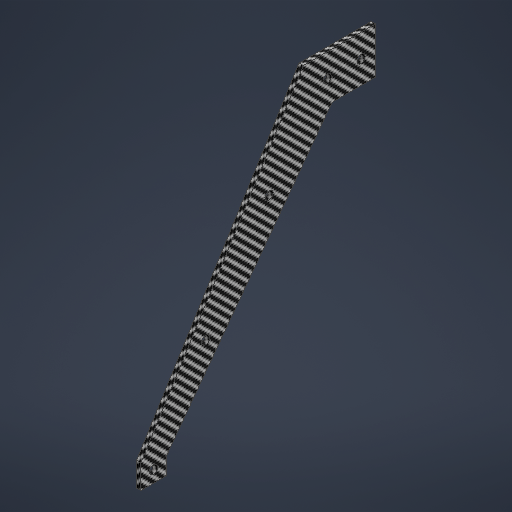
# Autodesk Inventor part: pata
Saved by Autodesk Inventor 2026.1 (Build 301233020, 233B)
## iProperties
Created: 2025-07-24
Part Number: pata
Material: Polímero reforzado con fibra de carbono
Document SubType Name: Modeling
Designer: rodri
Density: 1.43 g/cm^3
Appearance: Fibra de carbono
Author: rodri
Autodesk Inventor part; units mm, degrees
ref_plane "YZ Plane" through (0, 0, 0) normal (1, 0, 0) x (0, 1, 0)
ref_plane "XZ Plane" through (0, 0, 0) normal (0, 1, 0) x (-1, 0, 0)
ref_plane "XY Plane" through (0, 0, 0) normal (0, 0, 1) x (1, 0, 0)
sketch "Boceto1" plane through (0, 0, 0) normal (1, 0, 0) x (0, 1, 0)
  line L0 (9.583, -8.5639) -> (9.583, 60.4361) construction
  line L1 (9.583, -8.5639) -> (-83.417, -8.5639) construction
  line L2 (9.583, -8.5639) -> (-83.417, 60.4361)
  line L3 (-83.417, 60.4361) -> (-90.417, 60.4361)
  line L4 (-90.417, 60.4361) -> (-90.417, 70.9361)
  line L5 (-90.417, 70.9361) -> (-80.417, 70.9361)
  line L6 (9.583, -8.5639) -> (9.583, -26.5639)
  line L7 (9.583, -26.5639) -> (28.783, -26.5639)
  line L8 (28.783, -26.5639) -> (28.783, 3.4361)
  line L9 (-80.417, 70.9361) -> (28.783, 3.4361)
  line L10 (19.183, -26.5639) -> (19.183, 22.2031) construction
  line L11 (9.583, 30.9188) -> (-10.817, 30.9188) construction
  line L12 (9.583, 46.0673) -> (-49.717, 46.0673) construction
  line L13 (-90.417, 65.6861) -> (-76.0379, 65.6861) construction
  line L14 (-80.417, 70.9361) -> (-83.417, 60.4361) construction
  line L15 (28.783, 3.4361) -> (9.583, -8.5639) construction
  line L16 (-81.917, 65.6861) -> (19.183, -2.5639) construction
  point P0 (19.183, -20.5639)
  point P1 (19.183, -6.5639)
  point P2 (-85.417, 65.6861)
  point P3 (-49.717, 43.9487)
  point P4 (-10.817, 17.6883)
  dimension "d4" = 69
  dimension "d5" = 93
  dimension "d6" = 7
  dimension "d7" = 10.5
  dimension "d8" = 10
  dimension "d9" = 18
  dimension "d10" = 19.2
  dimension "d11" = 30
  dimension "d12" = 14
  dimension "d13" = 6
  dimension "d16" = 20.4
  dimension "d17" = 59.3
  dimension "d18" = 5
  constraints: 34 end point, 7 point on line, 4 horizontal, 4 midpoint, 4 perpendicular, 4 vertical
  measures "d4" distance of L0.start L0.end
  measures "d5" distance of L0.start L1.end
  measures "d6" distance of L2.end L3.end
  measures "d7" distance of L3.end L4.end
  measures "d8" distance of L4.end L5.end
  measures "d9" distance of L0.start L6.end
  measures "d10" distance of L6.end L7.end
  measures "d11" distance of L7.end L8.end
  measures "d12" distance of point (19.183, -6.564) point (19.183, -20.564)
  measures "d13" distance of point (19.183, -20.564) L10.start
  measures "d16" distance of L11.start L11.end
  measures "d17" distance of L12.start L12.end
  measures "d18" distance from line of point (-85.417, 65.686) L4
extrude "Extrusión1" add sketch "Boceto1" along normal blind 1.8
hole "Agujero1" at (0, 19.183, -20.5639) at (0, 19.183, -6.5639) at (0, -85.417, 65.6861) at (0, -49.717, 43.9487) at (0, -10.817, 17.6883) direction (1, 0, 0) diameter 3.4 end through all clearance for "Tornillo para maquinaria de cabeza plana" size "M3" standard "Perfil M métrico ANSI"
